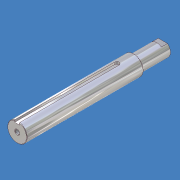
# Autodesk Inventor part: BB1-Axle
Saved by Autodesk Inventor 2015 (Build 190159000, 159)
## iProperties
Company: FirstCadLibrary
Shininess: 64.0
Length Units: 11269
Angle Units: 11279
Time Units: 11290
Mass Units: 11283
Length Display Precision: 3
Angle Display Precision: 2
Compacted: True
Part Number: BB1-Axle
Document SubType Name: Modeling
Created: 2007-01-08
Material: Steel, Mild
Designer: Ed Sparks
Catalog Web Link: www.banebots.com
Vendor: BaneBots
Density: 1 g/cm^3
Appearance: Metal-AL-6061 (Polished)
Density: 0.0
Volumn: 0.0
Area: 0.0
PropertySet Name: Model Information
Control State: 0
Master: False
Checked Out: False
Author: Ed Sparks
Autodesk Inventor part; units mm, degrees
ref_plane "YZ Plane" through (0, 0, 0) normal (1, 0, 0) x (0, 1, 0)
ref_plane "XZ Plane" through (0, 0, 0) normal (0, 1, 0) x (-1, 0, 0)
sketch "Sketch1" plane through (0, 0, 0) normal (0, 0, 1) x (1, 0, 0)
  circle A0 centre (0, 0) radius 6.35
  dimension "d0" = 12.7
  constraints: 1 centre point, 1 coincident, 1 other
  measures "d0" diameter of A0
extrude "Extrusion1" add sketch "Sketch1" along normal mid plane 76.2
sketch "Sketch2" plane through (0, 0, 38.1) normal (0, 0, 1) x (1, 0, 0)
  circle A0 centre (0, 0) radius 6.35 projected
  circle A1 centre (0, 0) radius 5
  dimension "d3" = 10
  constraints: 1 centre point, 1 coincident, 1 concentric
  measures "d3" diameter of A1
extrude "Extrusion2" add sketch "Sketch2" along normal blind 19 contours A1
sketch "Sketch3" plane through (0, 0, 57.1) normal (0, 0, 1) x (1, 0, 0)
  circle A0 centre (0, 0) radius 5 projected
  line L0 (-4, 3) -> (-4, -3)
  line L1 (4, 3) -> (4, -3)
  line L2 (4, 0) -> (5, 0) construction
  line L3 (-4, 0) -> (-5, 0) construction
  dimension "d7" = 8
  constraints: 8 end point, 6 point on circle, 2 collinear, 2 midpoint, 2 vertical, 1 perpendicular
  measures "d7" distance between parallel lines of L1 L0
extrude "Extrusion3" cut sketch "Sketch3" against normal blind 4 contours A0 L1 | L0 A0
sketch "Sketch4" plane through (0, 0, -38.1) normal (0, 0, -1) x (-1, 0, 0)
  circle A0 centre (0, 0) radius 6.35 projected
  constraints: 1 coincident
hole "Hole1" at (0, 0, -38.1) direction (0, 0, 1) diameter 2.85 depth 19 tip angle 118 thread size "M3.5x0.6" class "6H" standard "ANSI Metric M Profile"
chamfer "Chamfer1" distance 0.25 angle 45 3 edges at (0, -1.425, -38.1) (-6.35, 0, -38.1) (-6.35, 0, 38.1)
ref_plane "Work Plane1" through (-6.35, 0, 0) normal (1, 0, 0) x (0, 1, 0)
sketch "Sketch5" plane through (-6.35, 0, 0) normal (1, 0, 0) x (0, 1, 0)
  line L0 (6.1, -38.1) -> (-6.1, -38.1) projected
  line L1 (0, -38.1) -> (0, 22.7756) construction
  arc A0 (1.5875, 26.9) -> (-1.5875, 26.9) centre (0, 26.9) ccw
  line L2 (1.5875, -38.1) -> (1.5875, 26.9)
  line L3 (-1.5875, 26.9) -> (-1.5875, -38.1)
  dimension "d20" = 3.175
  dimension "d25" = 65
  constraints: 6 end point, 3 point on line, 2 parallel, 2 point on circle, 2 tangent, 1 centre point, 1 midpoint, 1 perpendicular
  measures "d20" distance between parallel lines of L3 L2
  measures "d25" distance from line of A0.centre L0
extrude "Extrusion4" cut sketch "Sketch5" along normal blind 1.5875
body "Solid1"
